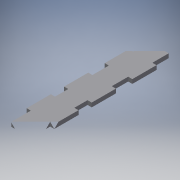
# Autodesk Inventor part: front
Saved by Autodesk Inventor 2016 (Build 200138000, 138)
## iProperties
Created: 2016-05-17
Part Number: front
Material: Generic
Document SubType Name: Modeling
Designer: Lillahunden
Density: 1 g/cm^3
Appearance: Default
Author: Lillahunden
Autodesk Inventor part; units mm, degrees
ref_plane "YZ Plane" through (0, 0, 0) normal (1, 0, 0) x (0, 1, 0)
ref_plane "XZ Plane" through (0, 0, 0) normal (0, 1, 0) x (-1, 0, 0)
ref_plane "XY Plane" through (0, 0, 0) normal (0, 0, 1) x (1, 0, 0)
sketch "Sketch1" plane through (0, 0, 0) normal (0, 0, 1) x (1, 0, 0)
  line L0 (0, 0) -> (0, -23.75)
  line L1 (0, -23.75) -> (6, -23.75)
  line L2 (6, 0) -> (6, -23.75)
  line L3 (0, 0) -> (6, 0)
  line L4 (0, -23.75) -> (0, -58.75)
  line L5 (0, -58.75) -> (6, -58.75)
  line L6 (6, -23.75) -> (6, -58.75) construction
  line L7 (0, -23.75) -> (6, -23.75)
  line L8 (0, -58.75) -> (0, -82.5)
  line L9 (0, -82.5) -> (6, -82.5)
  line L10 (6, -58.75) -> (6, -82.5)
  line L11 (0, -58.75) -> (6, -58.75)
  line L12 (0, -82.5) -> (0, -117.5)
  line L13 (0, -117.5) -> (6, -117.5)
  line L14 (6, -82.5) -> (6, -117.5) construction
  line L15 (0, -82.5) -> (6, -82.5)
  line L16 (0, -117.5) -> (0, -136.6283)
  line L17 (0, -136.6283) -> (6, -136.6283)
  line L18 (6, -117.5) -> (6, -136.6283)
  line L19 (0, -117.5) -> (6, -117.5)
  line L20 (0, -136.6283) -> (0, -171.6283)
  line L21 (0, -171.6283) -> (6, -171.6283)
  line L22 (6, -136.6283) -> (6, -171.6283) construction
  line L23 (0, -136.6283) -> (6, -136.6283)
  line L24 (0, -171.6283) -> (0, -200)
  line L25 (0, -200) -> (6, -200)
  line L26 (6, -171.6283) -> (6, -200)
  line L27 (0, -171.6283) -> (6, -171.6283)
  line L28 (0, -200) -> (40, -200)
  line L29 (40, -200) -> (40, 0)
  line L30 (40, 0) -> (0, 0)
  line L31 (0, 0) -> (0, -200)
extrude "Extrusion1" add sketch "Sketch1" against normal blind 6 contours L1 L2 L30 L29 L28 L26 L21 L20 L17 L18 L13 L12 L9 L10 L5 L4
sketch "Sketch2" plane through (0, 0, 0) normal (0, 0, 1) x (1, 0, 0)
  line L0 (6, 0) -> (6, -23.75) construction
  line L1 (6, -23.75) -> (0, -23.75) construction
  line L2 (0, -23.75) -> (0, -58.75) construction
  line L3 (0, -58.75) -> (6, -58.75) construction
  line L4 (6, -58.75) -> (6, -82.5) construction
  line L5 (0, -82.5) -> (6, -82.5) construction
  line L6 (0, -82.5) -> (0, -117.5) construction
  line L7 (0, -117.5) -> (6, -117.5) construction
  line L8 (6, -117.5) -> (6, -136.6283) construction
  line L9 (0, -136.6283) -> (6, -136.6283) construction
  line L10 (0, -136.6283) -> (0, -171.6283) construction
  line L11 (0, -171.6283) -> (6, -171.6283) construction
  line L12 (6, -171.6283) -> (6, -200) construction
  line L13 (40, 0) -> (40, -200) construction
  line L14 (40, -156.4035) -> (0, -156.4035) construction
  line L15 (0, -171.6283) -> (0, -136.6283) construction
  line L16 (20, -156.4035) -> (20, -119.6077) construction
  line L17 (34, 0) -> (34, -23.75)
  line L18 (34, -23.75) -> (40, -23.75)
  line L19 (40, -23.75) -> (40, -58.75)
  line L20 (40, -58.75) -> (34, -58.75)
  line L21 (34, -58.75) -> (34, -82.5)
  line L22 (40, -82.5) -> (34, -82.5)
  line L23 (40, -82.5) -> (40, -117.5)
  line L24 (40, -117.5) -> (34, -117.5)
  line L25 (34, -117.5) -> (34, -136.6283)
  line L26 (40, -136.6283) -> (34, -136.6283)
  line L27 (40, -136.6283) -> (40, -171.6283) construction
  line L28 (40, -171.6283) -> (34, -171.6283)
  line L29 (34, -171.6283) -> (34, -200)
  line L30 (0, -156.4035) -> (40, -156.4035) construction
  line L31 (40, -171.6283) -> (40, -136.6283) construction
  line L32 (40, 0) -> (40, -200) construction
  line L33 (40, -200) -> (6, -200) construction
  line L34 (34, -200) -> (40, -200)
  line L35 (6, 0) -> (40, 0) construction
  line L36 (34, 0) -> (40, 0)
  line L37 (40, -117.5) -> (40, -136.6283)
  line L38 (40, -171.6283) -> (40, -200)
  line L39 (40, 0) -> (40, -23.75)
  line L40 (40, -82.5) -> (40, -58.75)
  point P0 (0, 0)
  constraints: 32 end point, 16 symmetric about line, 7 collinear, 3 point on line, 1 midpoint, 1 perpendicular, 1 vertical
extrude "Extrusion2" cut sketch "Sketch2" against normal through all
body "Solid1"
